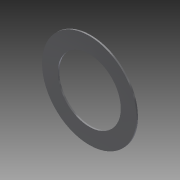
# Autodesk Inventor part: Thrust Washer .125 Thick 1.000 Shaft Diameter
Saved by Autodesk Inventor 2013 (Build 170138000, 138)
## iProperties
Created: 2013-04-02
Part Number: Thrust Washer .125 Thick 1.000 Shaft Diameter
Material: Generic
Document SubType Name: Modeling
Designer: mvarma
Density: 1 g/cm^3
Author: mvarma
Autodesk Inventor part; units mm, degrees
ref_plane "YZ Plane" through (0, 0, 0) normal (1, 0, 0) x (0, 1, 0)
ref_plane "XZ Plane" through (0, 0, 0) normal (0, 1, 0) x (-1, 0, 0)
ref_plane "XY Plane" through (0, 0, 0) normal (0, 0, 1) x (1, 0, 0)
sketch "Sketch1" plane through (0, 0, 0) normal (0, 0, 1) x (1, 0, 0)
  circle A0 centre (0, 0) radius 17.4625
  circle A1 centre (0, 0) radius 26.1938
  dimension "d0" = 34.925
  dimension "d2" = 52.3875
  constraints: 2 centre point, 2 coincident
  measures "d0" diameter of A0
  measures "d2" diameter of A1
extrude "Extrusion1" add sketch "Sketch1" along normal blind 0.7937
body "Solid1"
